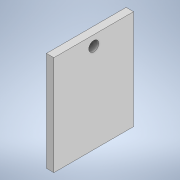
# Autodesk Inventor part: woodForAssemblyLeftSide
Saved by Autodesk Inventor 2021 (Build 250183000, 183)
## iProperties
Created: 2020-07-02
Part Number: woodForAssemblyLeftSide
Material: Generic
Document SubType Name: Modeling
Designer: robst
Density: 1 g/cm^3
Appearance: Default
Author: robst
Autodesk Inventor part; units mm, degrees
ref_plane "YZ Plane" through (0, 0, 0) normal (1, 0, 0) x (0, 1, 0)
ref_plane "XZ Plane" through (0, 0, 0) normal (0, 1, 0) x (-1, 0, 0)
ref_plane "Work Plane1" through (33.4366, -21.0953, -37.5679) normal (0, 1, 0) x (-1, 0, 0)
sketch "Sketch1" plane through (33.4366, -21.0953, -37.5679) normal (0, 1, 0) x (-1, 0, 0)
  line L0 (101.6, -101.6) -> (101.6, 101.6) projected
  line L1 (101.6, 101.6) -> (-101.6, 101.6) projected
  line L2 (-101.6, -101.6) -> (101.6, -101.6) projected
  line L3 (101.6, 101.6) -> (82.55, 101.6)
  line L4 (82.55, 101.6) -> (82.55, -101.6)
  line L5 (82.55, -101.6) -> (101.6, -101.6)
  line L6 (101.6, -101.6) -> (101.6, 101.6)
  point P0 (33.4366, 37.5679)
  dimension "d0" = 19.05
  constraints: 8 end point, 2 parallel, 1 horizontal, 1 perpendicular, 1 point on line
  measures "d0" distance between parallel lines of L4 L0
extrude "Extrusion1" add sketch "Sketch1" along normal blind 254
sketch "Sketch2" plane through (-68.1634, -21.0953, -139.1679) normal (-1, 0, 0) x (0, 0, 1)
  line L0 (203.2, 254) -> (0, 254) construction
  line L1 (101.6, 254) -> (101.6, 0) construction
  line L2 (203.2, 0) -> (0, 0) construction
  circle A0 centre (101.6, 228.6) radius 12.7
  point P0 (139.1679, 21.0953)
  dimension "d3" = 25.4
  dimension "d4" = 25.4
  constraints: 2 end point, 2 midpoint, 1 centre point, 1 point on line
  measures "d3" diameter of A0
  measures "d4" distance from line of A0.centre L0
extrude "Extrusion2" cut sketch "Sketch2" against normal through all
body "Solid1"
